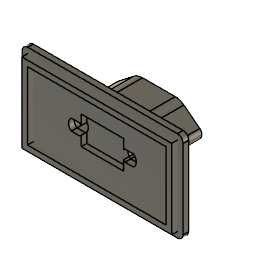
DD-fiche-v6 (Autodesk Fusion 360 design; units mm, degrees)
part number: 2025-12-20-11-26-56-309
Autodesk Fusion 360 part; units mm, degrees
sketch "Esquisse1" plane through (0, 0, 0) normal (0, 1, 0) x (1, 0, 0)
  circle A0 centre (10, -10) radius 2.5
  line L0 (8.5, -12) -> (11.5, -12)
  line L1 (8.5, -8) -> (11.5, -8)
  circle A1 centre (29, -10) radius 2.5
  line L2 (27.5, -12) -> (30.5, -12)
  line L3 (27.5, -8) -> (30.5, -8)
  line L4 (-8.9501, 6) -> (48.0499, 6)
  line L5 (48.0499, 6) -> (48.0499, -26)
  line L6 (48.0499, -26) -> (-8.9501, -26)
  line L7 (-8.9501, -26) -> (-8.9501, 6)
  line L8 (-7, -24) -> (46, -24)
  line L9 (46, -24) -> (46, 4)
  line L10 (46, 4) -> (-7, 4)
  line L11 (-7, 4) -> (-7, -24)
  line L12 (-5, -22) -> (44, -22)
  line L13 (44, -22) -> (44, 2)
  line L14 (44, 2) -> (-5, 2)
  line L15 (-5, 2) -> (-5, -22)
  line L16 (10, -12) -> (8.5, -12)
  line L17 (3, -10) -> (12, -17)
  line L18 (12, -17) -> (27, -17)
  line L19 (27, -17) -> (36, -10)
  line L20 (36, -10) -> (27, -3)
  line L21 (27, -3) -> (12, -3)
  line L22 (12, -3) -> (3, -10)
  line L23 (12, -15) -> (27, -15)
  line L24 (27, -15) -> (27, -5)
  line L25 (27, -5) -> (12, -5)
  line L26 (12, -5) -> (12, -15)
  constraint coincident A0 L0.start
  constraint coincident A0 L0.end
  constraint horizontal L0
  constraint coincident A0 L1.start
  constraint coincident A0 L1.end
  constraint parallel L0 L1
  constraint coincident A1 L2.start
  constraint coincident A1 L2.end
  constraint horizontal L2
  constraint coincident A1 L3.start
  constraint coincident A1 L3.end
  constraint parallel L2 L3
  constraint horizontal L4
  constraint vertical L5
  constraint horizontal L6
  constraint vertical L7
  constraint horizontal L8
  constraint vertical L9
  constraint horizontal L10
  constraint vertical L11
  constraint horizontal L12
  constraint vertical L13
  constraint horizontal L14
  constraint vertical L15
  constraint midpoint L0 L16.start
  constraint horizontal L18
  constraint parallel L17 L20
  constraint parallel L19 L22
  constraint perpendicular L24 L25
  constraint perpendicular L23 L26
extrude "Extrusion40" add sketch "Esquisse1" against normal blind 2 contours A0 L1 | A0 L0 L16 | A1 L3 | A1 L2 | L4 L5 L6 L7 | L8 L9 L10 L11 | L12 L13 L14 L15 | L17 L18 L19 L20 L21 L22 makes body 1
extrude "Extrusion41" add sketch "Esquisse1" against normal blind 4 separate body contours L8 L9 L10 L11 makes body 2
extrude "Extrusion42" add sketch "Esquisse1" along normal blind 18 separate body contours A0 L1 | A0 A1 L23 L24 L25 L26 | A0 L0 L16 | A1 L3 | A1 L2 | L17 L18 L19 L20 L21 L22 makes body 3
extrude "Extrusion43" add sketch "Esquisse1" along normal blind 12 separate body contours A0 A1 L23 L24 L25 L26 makes body 4
fillet "Congé11" radius 5 4 edges at (12, 9, 17) (27, 9, 17) (12, 9, 3) (27, 9, 3) on bodies 3
fillet "Congé12" radius 2 2 edges at (36, 9, 10) (3, 9, 10) on bodies 3
fillet "Congé13" radius 2 4 edges at (48.0499, -1, 26) (48.0499, -1, -6) (-8.9501, -1, -6) (-8.9501, -1, 26) on bodies 1
